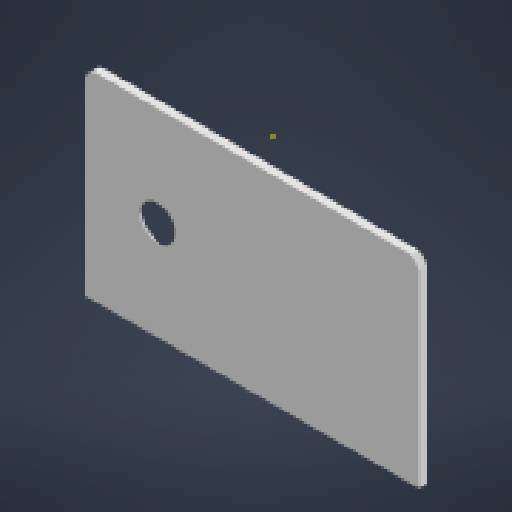
# Autodesk Inventor part: AASTRC Bottom case cover
Saved by Autodesk Inventor 2024 (Build 280153000, 153)
## iProperties
Created: 2023-07-16
Part Number: AASTRC Bottom case cover
Material: 일반
Document SubType Name: Modeling
Designer: 6gioc
Density: 1 g/cm^3
Appearance: 기본값
Mass: 130.356 g
Surface Area: 554.511 cm^2
Volume: 130.356 cm^3
Author: 6gioc
Autodesk Inventor part; units mm, degrees
ref_plane "YZ Plane" through (0, 0, 0) normal (1, 0, 0) x (0, 1, 0)
ref_plane "XZ Plane" through (0, 0, 0) normal (0, 1, 0) x (-1, 0, 0)
ref_plane "XY Plane" through (0, 0, 0) normal (0, 0, 1) x (1, 0, 0)
sketch "스케치1" plane through (0, 0, 0) normal (0, 0, 1) x (1, 0, 0)
  line L0 (92.7067, -147.2632) -> (-114.2933, -147.2632)
  line L1 (-114.2933, -147.2632) -> (-114.2933, -26.2632)
  line L2 (-109.2933, -21.2632) -> (87.7067, -21.2632)
  line L3 (92.7067, -26.2632) -> (92.7067, -147.2632)
  arc A0 (92.7067, -26.2632) -> (87.7067, -21.2632) centre (87.7067, -26.2632) ccw
  arc A1 (-109.2933, -21.2632) -> (-114.2933, -26.2632) centre (-109.2933, -26.2632) ccw
  point P0 (0, 0)
  point P1 (-114.2933, -21.2632)
  point P2 (92.7067, -21.2632)
  dimension "d0" = 207
  dimension "d1" = 126
  dimension "d10" = 5
  constraints: 8 end point, 4 point on circle, 4 point on line, 4 tangent, 2 centre point, 2 parallel, 1 equal radius, 1 horizontal, 1 perpendicular
  measures "d0" distance of point (-114.293, -21.263) point (92.707, -21.263)
  measures "d1" distance of point (92.707, -21.263) L0.start
  measures "d10" radius of A0
extrude "돌출1" add sketch "스케치1" along normal blind 5
sketch "스케치2" plane through (0, 0, 5) normal (0, 0, 1) x (1, 0, 0)
  point P0 (0, 0)
